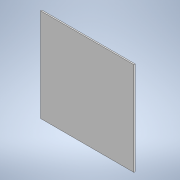
# Autodesk Inventor part: CaseBottom
Saved by Autodesk Inventor 2020.1 (Build 241239000, 239)
## iProperties
Created: 2019-09-03
Part Number: CaseBottom
Material: Generic
Document SubType Name: Modeling
Designer: matteo.spadetto-1
Density: 1 g/cm^3
Appearance: Default
Author: matteo.spadetto-1
Autodesk Inventor part; units mm, degrees
ref_plane "YZ Plane" through (0, 0, 0) normal (1, 0, 0) x (0, 1, 0)
ref_plane "XZ Plane" through (0, 0, 0) normal (0, 1, 0) x (-1, 0, 0)
ref_plane "XY Plane" through (0, 0, 0) normal (0, 0, 1) x (1, 0, 0)
sketch "Sketch1" plane through (0, 0, 0) normal (0, 0, 1) x (1, 0, 0)
  line L0 (0, 0) -> (65, 0)
  line L1 (65, 0) -> (65, 65)
  line L2 (65, 65) -> (0, 65)
  line L3 (0, 65) -> (0, 0)
  dimension "d0" = 65
  dimension "d1" = 65
  constraints: 8 end point, 2 parallel, 1 horizontal, 1 perpendicular
  measures "d0" distance of L2.end L1.end
  measures "d1" distance of L1.end L0.end
extrude "Extrusion1" add sketch "Sketch1" along normal blind 2.3
sketch "Sketch2" plane through (0, 0, 2.3) normal (0, 0, 1) x (1, 0, 0)
  line L0 (-4, 69) -> (69, 69)
  line L1 (69, 69) -> (69, -4)
  line L2 (69, -4) -> (-4, -4)
  line L3 (-4, -4) -> (-4, 69)
  point P0 (0, 0)
  point P1 (0, 65)
  point P2 (65, 0)
  constraints: 8 end point, 2 parallel, 1 perpendicular
extrude "Extrusion2" add sketch "Sketch2" along normal blind 1
sketch "Sketch3" plane through (0, 0, 0) normal (0, 0, -1) x (-1, 0, 0)
  line L0 (0, 0) -> (-65, 0) projected
  line L1 (0, 65) -> (0, 0) projected
  line L2 (-65, 0) -> (-65, 65) projected
  line L3 (-52, 65) -> (-52, 26)
  line L4 (-52, 26) -> (0, 26)
  line L5 (-51, 27) -> (-51, 65)
  line L6 (-51, 65) -> (-52, 65)
  line L7 (0, 65) -> (-1, 65)
  line L8 (-51, 27) -> (0, 27)
  point P0 (0, 26)
  constraints: 12 end point, 3 perpendicular, 1 horizontal, 1 parallel, 1 point on line
extrude "Extrusion5" add sketch "Sketch3" along normal blind 1
sketch "Sketch6" plane through (0, 0, 0) normal (0, 0, -1) x (-1, 0, 0)
  line L0 (-65, 65) -> (-52, 65) projected
  line L1 (-65, 55.5) -> (-52, 55.5)
  line L2 (-52, 26) -> (-52, 65) projected
  line L3 (-52, 55.5) -> (-52, 9.5)
  line L4 (-52, 9.5) -> (-65, 9.5)
  line L5 (-65, 9.5) -> (-65, 55.5)
  line L6 (-65, 0) -> (-65, 65) projected
  point P0 (0, 0)
  dimension "d23" = 46
  constraints: 8 end point, 2 collinear, 1 point on line
  measures "d23" distance of L1.end L3.end
extrude "Extrusion6" cut sketch "Sketch6" against normal blind 3 contours L1 L2 L3 L4 L5
sketch "Sketch7" plane through (0, 0, 0) normal (0, 0, -1) x (-1, 0, 0)
  line L0 (-65, 9.5) -> (-65, 55.5) projected
  line L1 (-52, 55.5) -> (-52, 65) projected
  line L2 (-52, 55.5) -> (-65, 55.5)
  line L3 (-65, 55.5) -> (-65, 58.5)
  line L4 (-65, 58.5) -> (-52, 58.5)
  line L5 (-52, 58.5) -> (-52, 55.5)
  point P0 (0, 0)
  constraints: 8 end point, 2 parallel, 1 horizontal, 1 perpendicular
extrude "Extrusion7" cut sketch "Sketch7" against normal blind 3
sketch "Sketch8" plane through (0, 0, 0) normal (0, 0, -1) x (-1, 0, 0)
  line L0 (-52, 26) -> (-52, 9.5) projected
  line L1 (-52, 26) -> (-52, 0)
  line L2 (-52, 26) -> (-51, 26)
  line L3 (-51, 26) -> (-51, 0)
  line L4 (0, 0) -> (-65, 0) projected
  line L5 (-52, 0) -> (-51, 0)
  line L6 (-51, 26) -> (-33, 26)
  line L7 (0, 26) -> (-52, 26) projected
  line L8 (-33, 26) -> (-33, 0)
  line L9 (-33, 0) -> (-32, 0)
  line L10 (-32, 0) -> (-32, 26)
  line L11 (-32, 26) -> (-33, 26)
  dimension "d32" = 1
  constraints: 18 end point, 5 point on line, 4 perpendicular, 1 collinear, 1 horizontal, 1 vertical
  measures "d32" distance of L8.end L9.end
extrude "Extrusion8" add sketch "Sketch8" along normal blind 1 contours L2 L3 L4 L1 L0 | L7 L10 L4 L8
sketch "Sketch9" plane through (0, 0, 0) normal (0, 0, -1) x (-1, 0, 0)
  line L0 (0, 26) -> (0, 0) projected
  line L1 (0, 26) -> (-32, 26) projected
  line L2 (-2, 26) -> (-12, 26)
  line L3 (-12, 26) -> (-12, 14)
  line L4 (-12, 14) -> (-2, 14)
  line L5 (-2, 14) -> (-2, 26)
  line L6 (-1, 13) -> (-13, 13)
  line L7 (-13, 13) -> (-13, 26)
  line L8 (-1, 13) -> (-1, 26)
  line L9 (-12, 26) -> (-13, 26)
  line L10 (-2, 26) -> (-1, 26)
  dimension "d35" = 2
  dimension "d36" = 10
  dimension "d37" = 12
  constraints: 18 end point, 4 perpendicular, 4 point on line, 2 collinear, 1 parallel
  measures "d35" distance of L0.start L2.start
  measures "d36" distance of L2.start L2.end
  measures "d37" distance of L2.end L3.end
extrude "Extrusion9" add sketch "Sketch9" along normal blind 1 contours L8 L6 L7 L1 L3 L4 L5
sketch "Sketch12" plane through (0, 0, 0) normal (0, 0, -1) x (-1, 0, 0)
  line L0 (-12, 14) -> (-2, 14) projected
  line L1 (-12, 26) -> (-2, 26) projected
  line L2 (-12, 14) -> (-2, 14)
  line L3 (-2, 14) -> (-2, 26)
  line L4 (-2, 26) -> (-12, 26)
  line L5 (-12, 26) -> (-12, 14)
  point P0 (0, 0)
  constraints: 8 end point, 2 parallel, 1 horizontal, 1 perpendicular
extrude "Extrusion11" cut sketch "Sketch12" against normal blind 3
fillet "Fillet1" radius 6.5 2 edges at (7, 14, 3) (7, 26, 3)
body "Solid1"
